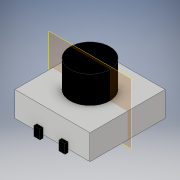
# Autodesk Inventor part: Push_Button
Saved by Autodesk Inventor 2019.4 (Build 234330000, 330)
## iProperties
Created: 2021-06-27
Part Number: Push_Button
Material: Generic
Document SubType Name: Modeling
Designer: keshav
Density: 1 g/cm^3
Appearance: Default
Author: keshav
Autodesk Inventor part; units mm, degrees
ref_plane "YZ Plane" through (0, 0, 0) normal (1, 0, 0) x (0, 1, 0)
ref_plane "XZ Plane" through (0, 0, 0) normal (0, 1, 0) x (-1, 0, 0)
sketch "Sketch1" plane through (0, 0, 0) normal (0, 1, 0) x (-1, 0, 0)
  line L0 (-6, 6) -> (6, 6)
  line L1 (6, 6) -> (6, -6)
  line L2 (6, -6) -> (-6, -6)
  line L3 (-6, -6) -> (-6, 6)
  line L4 (-6, 6) -> (6, -6) construction
  line L5 (6, 6) -> (-6, -6) construction
  point P0 (0, 0)
  dimension "d0" = 12
  dimension "d1" = 12
  constraints: 12 end point, 2 midpoint, 2 parallel, 1 horizontal, 1 perpendicular
  measures "d0" distance of L1.end L2.end
  measures "d1" distance of L0.end L1.end
extrude "Extrusion1" add sketch "Sketch1" along normal blind 4
sketch "Sketch2" plane through (0, 4, 0) normal (0, 1, 0) x (1, 0, 0)
  circle A0 centre (0, 0) radius 3.175
  dimension "d4" = 6.35
  constraints: 1 centre point, 1 coincident
  measures "d4" diameter of A0
extrude "Extrusion2" add sketch "Sketch2" along normal blind 4.35
sketch "Sketch3" plane through (-6, 0, 6) normal (0, 0, 1) x (1, 0, 0)
  line L0 (3.5, 1) -> (4.5, 1)
  line L1 (4.5, 1) -> (4.5, -0.5)
  line L2 (12, 0) -> (0, 0) projected
  line L3 (4.5, -0.5) -> (3.5, -0.5)
  line L4 (3.5, -0.5) -> (3.5, 1)
  line L5 (0, 0) -> (0, 4) projected
  line L6 (6, 3.8576) -> (6, 0) construction
  line L7 (8.5, 1) -> (7.5, 1)
  line L8 (7.5, 1) -> (7.5, -0.5)
  line L9 (7.5, -0.5) -> (8.5, -0.5)
  line L10 (8.5, -0.5) -> (8.5, 1)
  dimension "d7" = 1
  dimension "d8" = 1
  dimension "d9" = 1.5
  dimension "d10" = 3.5
  constraints: 18 end point, 4 symmetric about line, 3 perpendicular, 2 horizontal
  measures "d7" distance of L0.end L0.start
  measures "d8" distance between parallel lines of L2 L0
  measures "d9" distance of L1.end L0.end
  measures "d10" distance between parallel lines of L5 L4
extrude "Extrusion3" add sketch "Sketch3" along normal blind 0.5
mirror "Mirror1" about plane through (0, 0, 0) normal (0, 0, 1) of "Extrusion3"
body "Solid1"
